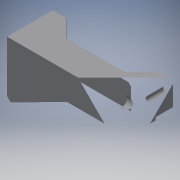
# Autodesk Inventor part: Crossmount
Saved by Autodesk Inventor 2016 (Build 200138000, 138)
## iProperties
Created: 2016-07-16
Part Number: Crossmount
Material: Generic
Document SubType Name: Modeling
Designer: Scott
Density: 1 g/cm^3
Appearance: Default
Author: Scott
Autodesk Inventor part; units mm, degrees
ref_plane "YZ Plane" through (0, 0, 0) normal (1, 0, 0) x (0, 1, 0)
ref_plane "XZ Plane" through (0, 0, 0) normal (0, 1, 0) x (-1, 0, 0)
ref_plane "XY Plane" through (0, 0, 0) normal (0, 0, 1) x (1, 0, 0)
sketch "Sketch1" plane through (0, 0, 0) normal (0, 0, 1) x (1, 0, 0)
  circle A0 centre (0, 0) radius 4 projected
  circle A1 centre (-152.4, 0) radius 4 projected
  circle A2 centre (0, 0) radius 10.16
  circle A3 centre (-152.4, 0) radius 10.16
  point P0 (0, 0)
  dimension "d0" = 20.32
  dimension "d1" = 20.32
  constraints: 2 centre point, 2 coincident
  measures "d0" diameter of A2
  measures "d1" diameter of A3
extrude "Extrusion1" add sketch "Sketch1" against normal blind 25.4
sketch "Sketch2" plane through (0, 0, 0) normal (0, 0, 1) x (1, 0, 0)
  circle A0 centre (-152.4, 0) radius 10.16 projected
  circle A1 centre (0, 0) radius 10.16 projected
  line L0 (10.16, -10.16) -> (-162.56, -10.16)
  line L1 (-162.56, -10.16) -> (-162.56, 10.16)
  line L2 (-162.56, 10.16) -> (10.16, 10.16)
  line L3 (10.16, 10.16) -> (10.16, -10.16)
  point P0 (0, 0)
  constraints: 8 end point, 2 parallel, 1 horizontal, 1 perpendicular
extrude "Extrusion2" add sketch "Sketch2" along normal blind 38.1
sketch "Sketch3" plane through (-162.56, -10.16, 0) normal (-1, 0, 0) x (0, 0, 1)
  circle A0 centre (18.605, 8.132) radius 4 projected
  line L0 (-0.445, -10.918) -> (37.655, -10.918)
  line L1 (37.655, -10.918) -> (37.655, 27.182)
  line L2 (37.655, 27.182) -> (-0.445, 27.182)
  line L3 (-0.445, 27.182) -> (-0.445, -10.918)
  line L4 (-0.445, -10.918) -> (37.655, 27.182) construction
  line L5 (37.655, -10.918) -> (-0.445, 27.182) construction
  point P0 (0, 10.16)
  dimension "d6" = 38.1
  dimension "d7" = 38.1
  constraints: 12 end point, 2 midpoint, 2 parallel, 1 horizontal, 1 perpendicular
  measures "d6" distance of L2.end L1.end
  measures "d7" distance of L1.end L0.end
extrude "Extrusion3" add sketch "Sketch3" against normal up to surface (172.72 mm away)
sketch "Sketch4" plane through (-162.56, -10.16, 38.1) normal (-1, 0, 0) x (0, 0, 1)
  circle A0 centre (-19.495, 8.132) radius 4 projected
  circle A1 centre (-19.495, 8.132) radius 11
  point P0 (-38.1, 10.16)
  dimension "d10" = 22
  constraints: 1 centre point, 1 coincident
  measures "d10" diameter of A1
extrude "Extrusion4" cut sketch "Sketch4" against normal blind 7 contours A0 | A1
sketch "Sketch5" plane through (-155.56, -2.028, 18.605) normal (-1, 0, 0) x (0, 0, 1)
  circle A0 centre (0, 0) radius 5 projected
  point P0 (-18.605, 2.028)
extrude "Extrusion5" cut sketch "Sketch5" against normal blind 214.9625
sketch "Sketch6" plane through (10.16, -10.16, 38.1) normal (1, 0, 0) x (0, 0, -1)
  circle A0 centre (19.495, 8.132) radius 5 projected
  line L0 (0.445, 20.32) -> (0, 20.32) projected
  line L1 (0, 0) -> (0, 20.32) projected
  line L2 (0.445, 0) -> (0, 0) projected
  line L3 (0.445, -10.918) -> (0.445, 0) projected
  line L4 (38.545, -10.918) -> (0.445, -10.918) projected
  line L5 (38.545, 10.16) -> (38.545, -10.918) projected
  line L6 (38.545, 27.182) -> (38.545, 10.16) projected
  line L7 (0.445, 27.182) -> (38.545, 27.182) projected
  line L8 (0.445, 20.32) -> (0.445, 27.182) projected
  circle A1 centre (19.495, 8.132) radius 11
  point P0 (38.1, 10.16)
  dimension "d15" = 22
  constraints: 1 centre point, 1 coincident
  measures "d15" diameter of A1
extrude "Extrusion6" cut sketch "Sketch6" against normal blind 7 contours A1
sketch "Sketch7" plane through (0, 0, -25.4) normal (0, 0, -1) x (-1, 0, 0)
  line L0 (-10.16, 17.022) -> (-10.16, 0) projected
  circle A0 centre (0, 0) radius 10.16 projected
  line L1 (-10.16, 0) -> (-10.16, -21.078) projected
  line L2 (162.56, -21.078) -> (-10.16, -21.078) projected
  line L3 (162.56, 0) -> (162.56, -21.078) projected
  circle A1 centre (152.4, 0) radius 10.16 projected
  line L4 (162.56, 17.022) -> (162.56, 0) projected
  line L5 (162.56, 17.022) -> (-10.16, 17.022) projected
  line L6 (162.56, 17.022) -> (-10.16, 17.022) projected
  line L7 (-10.16, -17.022) -> (10.16, -17.022)
  line L8 (10.16, -17.022) -> (10.16, 17.022)
  line L9 (10.16, 17.022) -> (-10.16, 17.022)
  line L10 (-10.16, 17.022) -> (-10.16, -17.022)
  line L11 (-10.16, -17.022) -> (10.16, 17.022) construction
  line L12 (10.16, -17.022) -> (-10.16, 17.022) construction
  point P0 (0, 0)
  constraints: 12 end point, 2 horizontal alignment, 2 midpoint, 2 parallel, 1 horizontal, 1 perpendicular, 1 point on line
extrude "Extrusion7" add sketch "Sketch7" against normal up to surface (24.955 mm away) contours L5 L8 A0 L0 | A0 L8 L7 L1
chamfer "Chamfer1" distance 24.892 angle 45 1 edges at (-10.16, 0, -0.445)
sketch "Sketch8" plane through (-152.4, 0, -25.4) normal (0, 0, -1) x (-1, 0, 0)
  circle A0 centre (0, 0) radius 4 projected
  circle A1 centre (0, 0) radius 10.16 projected
  line L0 (-117.348, -17.022) -> (-117.348, 17.022) projected
  line L1 (-117.348, -17.022) -> (-162.56, -17.022) projected
  line L2 (-162.56, -17.022) -> (-162.56, -21.078) projected
  line L3 (10.16, -21.078) -> (-162.56, -21.078) projected
  line L4 (10.16, 0) -> (10.16, -21.078) projected
  circle A2 centre (0, 0) radius 10.16 projected
  line L5 (10.16, 17.022) -> (10.16, 0) projected
  line L6 (10.16, 17.022) -> (-117.348, 17.022) projected
  line L7 (10.16, -17.022) -> (-10.16, -17.022)
  line L8 (-10.16, -17.022) -> (-10.16, 17.022)
  line L9 (-10.16, 17.022) -> (10.16, 17.022)
  line L10 (10.16, 17.022) -> (10.16, -17.022)
  line L11 (10.16, -17.022) -> (-10.16, 17.022) construction
  line L12 (-10.16, -17.022) -> (10.16, 17.022) construction
  point P0 (-152.4, 0)
  constraints: 12 end point, 2 midpoint, 2 parallel, 1 horizontal, 1 horizontal alignment, 1 perpendicular, 1 point on line
extrude "Extrusion8" add sketch "Sketch8" against normal up to surface (24.955 mm away) contours L4 L7 L8 A1 | A1 L8 L6 L5
chamfer "Chamfer2" distance 24.892 angle 45 1 edges at (-142.24, 0, -0.445)
sketch "Sketch9" plane through (-155.56, -2.028, 18.605) normal (-1, 0, 0) x (0, 0, 1)
  circle A0 centre (0, 0) radius 11 projected
  circle A1 centre (0, 0) radius 7.5
  point P0 (-18.605, 2.028)
  dimension "d28" = 15
  constraints: 1 centre point, 1 coincident
  measures "d28" diameter of A1
extrude "Extrusion9" cut sketch "Sketch9" against normal blind 219.725 contours A1
sketch "Sketch10" plane through (-162.56, -10.16, 38.1) normal (-1, 0, 0) x (0, 0, 1)
  circle A0 centre (-19.495, 8.132) radius 11 projected
  line L0 (-0.445, 0) -> (0, 0) projected
  line L1 (0, 20.32) -> (0, 0) projected
  line L2 (-0.445, 20.32) -> (0, 20.32) projected
  line L3 (-0.445, 20.32) -> (-0.445, 27.182) projected
  line L4 (-0.445, 27.182) -> (-63.5, 27.182) projected
  line L5 (-63.5, -6.862) -> (-63.5, 27.182) projected
  line L6 (-63.5, -6.862) -> (-38.545, -6.862) projected
  line L7 (-38.545, -6.862) -> (-38.545, -10.918) projected
  line L8 (-38.545, -10.918) -> (-0.445, -10.918) projected
  line L9 (-0.445, -10.918) -> (-0.445, 0) projected
  line L10 (-0.445, -10.918) -> (-41.445, -10.918)
  line L11 (-41.445, -10.918) -> (-41.445, -51.918)
  line L12 (-41.445, -51.918) -> (-0.445, -51.918)
  line L13 (-0.445, -51.918) -> (-0.445, -10.918)
  circle A1 centre (-20.945, -31.418) radius 12.5
  line L14 (-20.945, -31.418) -> (-20.945, -46.918)
  line L15 (-20.945, -46.918) -> (-5.445, -46.918)
  circle A2 centre (-5.445, -46.918) radius 2
  circle A3 centre (-36.445, -46.918) radius 2
  circle A4 centre (-5.445, -15.918) radius 2
  circle A5 centre (-36.445, -15.918) radius 2
  point P0 (-38.1, 10.16)
  dimension "d31" = 41
  dimension "d32" = 41
  dimension "d33" = 25
  dimension "d34" = 15.5
  dimension "d35" = 15.5
  dimension "d36" = 4
  dimension "d39" = 31
  dimension "d42" = 31
  constraints: 12 end point, 5 centre point, 3 parallel, 2 horizontal, 2 vertical, 1 coincident, 1 perpendicular, 6 other
  measures "d31" distance of L12.end L11.end
  measures "d32" distance of L11.end L10.end
  measures "d33" diameter of A1
  measures "d34" distance of L14.start L14.end
  measures "d35" distance of L14.end L15.end
  measures "d36" diameter of A2
  measures "d39" distance of A2.centre A3.centre
  measures "d42" distance of A2.centre A4.centre
extrude "Extrusion10" add sketch "Sketch10" against normal blind 5.08 contours L13 L12 L11 L10 L8
sketch "Sketch11" plane through (-162.56, -10.16, 37.655) normal (0, 0, 1) x (1, 0, 0)
  line L0 (0, 0) -> (172.72, 0) projected
  line L1 (0, -51.918) -> (0, 0) projected
  line L2 (0, -51.918) -> (5.08, -51.918) projected
  line L3 (5.08, -10.918) -> (5.08, -51.918) projected
  line L4 (5.08, -10.918) -> (172.72, -10.918) projected
  line L5 (172.72, -10.918) -> (172.72, 0) projected
  line L6 (0, -51.918) -> (5.08, -51.918) projected
  line L7 (5.08, -51.918) -> (86.36, -10.918)
  line L8 (5.08, -10.918) -> (172.72, -10.918) projected
  line L9 (86.36, -10.918) -> (172.72, -10.918)
  line L10 (172.72, 20.32) -> (172.72, 27.182) projected
  line L11 (172.72, -10.918) -> (172.72, 27.182)
  line L12 (172.72, 27.182) -> (0, 27.182)
  line L13 (0, -10.918) -> (0, -51.918) projected
  line L14 (0, 27.182) -> (0, -51.918)
  line L15 (5.08, -10.918) -> (5.08, -51.918) projected
  line L16 (0, -51.918) -> (5.08, -51.918)
  point P0 (162.56, 10.16)
  constraints: 12 end point, 4 perpendicular, 1 horizontal, 1 point on line
extrude "Extrusion11" add sketch "Sketch11" along normal blind 2.54
sketch "Sketch12" plane through (-157.48, -21.078, -0.445) normal (0, -1, 0) x (1, 0, 0)
  line L0 (0, 38.1) -> (0, 0) projected
  line L1 (0, 0) -> (167.64, 0) projected
  line L2 (167.64, 0) -> (167.64, 40.64) projected
  line L3 (81.28, 40.64) -> (167.64, 40.64) projected
  line L4 (81.28, 38.1) -> (81.28, 40.64) projected
  line L5 (0, 38.1) -> (81.28, 38.1) projected
  line L6 (167.64, 30.05) -> (167.64, 8.05) projected
  line L7 (167.64, 19.05) -> (-5.08, 18.87)
  line L8 (-5.08, -2.9) -> (-5.08, 40.64) projected
  line L9 (24.13, 31.66) -> (138.43, 31.66)
  line L10 (138.43, 31.66) -> (138.43, 6.26)
  line L11 (138.43, 6.26) -> (24.13, 6.26)
  line L12 (24.13, 6.26) -> (24.13, 31.66)
  line L13 (24.13, 31.66) -> (138.43, 6.26) construction
  line L14 (138.43, 31.66) -> (24.13, 6.26) construction
  point P0 (157.48, 0.445)
  point P1 (81.28, 18.96)
  dimension "d49" = 114.3
  dimension "d50" = 25.4
  constraints: 14 end point, 5 midpoint, 2 parallel, 1 horizontal, 1 perpendicular
  measures "d49" distance of L10.end L11.end
  measures "d50" distance of L9.end L10.end
extrude "Extrusion12" cut sketch "Sketch12" against normal blind 34.29 contours L12 L9 L10 L7 | L7 L10 L11 L12
sketch "Sketch13" plane through (-162.56, -62.078, -3.345) normal (0, 0, -1) x (-1, 0, 0)
  line L0 (0, 41) -> (0, 0) projected
  line L1 (0, 41) -> (-5.08, 41) projected
  line L2 (-5.08, 0) -> (-5.08, 41) projected
  line L3 (0, 0) -> (-5.08, 0) projected
  line L4 (-45.212, 79.1) -> (-45.212, 45.056) projected
  line L5 (-45.212, 79.1) -> (-127.508, 79.1) projected
  line L6 (-127.508, 45.056) -> (-127.508, 79.1) projected
  line L7 (-127.508, 45.056) -> (-172.72, 45.056) projected
  line L8 (-172.72, 45.056) -> (-172.72, 41) projected
  line L9 (-5.08, 41) -> (-172.72, 41) projected
  line L10 (0, 41) -> (-5.08, 41) projected
  line L11 (0, 45.056) -> (0, 41) projected
  line L12 (0, 45.056) -> (-45.212, 45.056) projected
  line L13 (-5.08, 0) -> (-5.08, 41) projected
  line L14 (-5.08, 0) -> (-38.8543, 45.056)
  point P0 (-162.56, 62.078)
  constraints: 2 end point, 1 point on line
extrude "Extrusion13" add sketch "Sketch13" along normal blind 2.54 contours L0 L3 L2 L1 | L1 L9 L14 L12 L11 | L2 L14 L9
body "Solid1"
